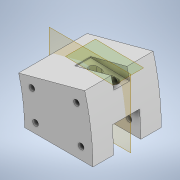
# Autodesk Inventor part: load_cell_mounting_block2
Saved by Autodesk Inventor 2022 (Build 260153000, 153)
## iProperties
Created: 2022-02-24
Part Number: load_cell_mounting_block2
Material: Generic
Document SubType Name: Modeling
Designer: Martijn
Density: 1 g/cm^3
Appearance: Default
Author: Martijn
Autodesk Inventor part; units mm, degrees
ref_plane "YZ Plane" through (0, 0, 0) normal (1, 0, 0) x (0, 1, 0)
ref_plane "XZ Plane" through (0, 0, 0) normal (0, 1, 0) x (-1, 0, 0)
ref_plane "XY Plane" through (0, 0, 0) normal (0, 0, 1) x (1, 0, 0)
sketch "Sketch1" plane through (0, 0, 0) normal (0, 0, 1) x (1, 0, 0)
  arc A0 (75, 0) -> (72.4444, 19.4114) centre (0, 0) ccw
  arc A1 (105, 0) -> (101.4222, 27.176) centre (0, 0) ccw
  line L0 (105, 0) -> (75, 0)
  line L1 (72.4444, 19.4114) -> (101.4222, 27.176)
  line L2 (75, 0) -> (0, 0)
  line L3 (0, 0) -> (72.4444, 19.4114)
  circle A2 centre (78.2518, 16.6329) radius 1.25
  circle A3 centre (79.8904, 4.1869) radius 1.25
  circle A4 centre (97.8148, 20.7912) radius 1.25
  circle A5 centre (99.863, 5.2336) radius 1.25
  line L4 (0, 0) -> (78.2518, 16.6329)
  line L5 (78.2518, 16.6329) -> (97.8148, 20.7912)
  line L6 (99.863, 5.2336) -> (79.8904, 4.1869)
  line L7 (79.8904, 4.1869) -> (0, 0)
  dimension "d0" = 20
  dimension "d1" = 15
  dimension "d2" = 3
  dimension "d3" = 3
  dimension "d4" = 2.5
  dimension "d5" = 80
  dimension "d6" = 75
  dimension "d7" = 105
  dimension "d8" = 80
  dimension "d9" = 20
  constraints: 16 end point, 6 centre point, 4 point on circle, 3 collinear, 3 equal radius, 2 coincident, 2 horizontal
  measures "d0" distance of L5.end L4.end
  measures "d1" angle of L0 L1
  measures "d2" angle of L1 L4
  measures "d3" angle of L0 L6
  measures "d4" diameter of A2
  measures "d5" distance of point (0, 0) L4.end
  measures "d6" radius of A0
  measures "d7" radius of A1
  measures "d8" distance of point (0, 0) L6.end
  measures "d9" distance of L6.end L6.start
extrude "Extrusion1" add sketch "Sketch1" along normal blind 30 contours A0 L1 A1 L0
ref_plane "Work Plane1" through (0, 0, 15) normal (0, 0, 1) x (1, 0, 0)
sketch "Sketch2" plane through (0, 0, 15) normal (0, 0, 1) x (1, 0, 0)
  line L0 (75, 0) -> (105, 0) projected
  line L1 (75, 0) -> (0, 0)
  line L2 (0, 0) -> (189.2794, -3.3039)
  line L3 (84.9871, -1.4835) -> (85.214, 11.5165)
  line L4 (85.214, 11.5165) -> (105.2109, 11.1675)
  line L5 (105.2109, 11.1675) -> (104.984, -1.8325)
  dimension "d12" = 13
  dimension "d13" = 1
  dimension "d14" = 85
  dimension "d15" = 105
  constraints: 10 end point, 2 parallel, 2 point on line, 1 horizontal, 1 perpendicular
  measures "d12" vertical distance of L3.start L3.end
  measures "d13" angle of L2 L0
  measures "d14" distance from line of L1.end L3
  measures "d15" distance from line of L5 L1.end
extrude "Extrusion2" cut sketch "Sketch2" along normal mid plane 12 contours L3 L4 L5 L2
sketch "Sketch3" plane through (104.4029, 11.1816, 9) normal (-0.0174524, -0.9998477, 0) x (0.9998477, -0.0174524, 0)
  arc A0 (-5, 4.3) -> (-5, 7.7) centre (-5, 6) ccw
  arc A1 (-7, 7.7) -> (-7, 4.3) centre (-7, 6) ccw
  line L0 (-7, 7.7) -> (-5, 7.7)
  line L1 (-5, 4.3) -> (-7, 4.3)
  line L2 (-19.1919, 12) -> (0.7921, 12) projected
  line L3 (0, 12) -> (0, 0) projected
  point P0 (-104.1919, -9)
  dimension "d19" = 3.4
  dimension "d20" = 6
  dimension "d21" = 5
  dimension "d22" = 2
  constraints: 4 end point, 4 point on circle, 4 tangent, 2 centre point, 2 horizontal
  measures "d19" distance between parallel lines of L1 L0
  measures "d20" distance from line of L2 A0.centre
  measures "d21" distance from line of L3 A0.centre
  measures "d22" distance of A0.centre A1.centre
extrude "Extrusion3" cut sketch "Sketch3" against normal blind 20
pattern_linear "Rectangular Pattern1" count 2 spacing 7.5 along (-0.9998477, 0.0174524, 0) of "Extrusion3"
ref_plane "Work Plane2" through (104.6822, 27.1792, 9) normal (-0.0174524, -0.9998477, 0) x (0.9998477, -0.0174524, 0)
sketch "Sketch5" plane through (104.6822, 27.1792, 9) normal (-0.0174524, -0.9998477, 0) x (0.9998477, -0.0174524, 0)
  line L0 (-19.0973, 2.5) -> (0.9027, 2.5)
  line L1 (0.9027, 2.5) -> (0.9027, 9.5)
  line L2 (0.9027, 9.5) -> (-19.0973, 9.5)
  line L3 (-19.0973, 9.5) -> (-19.0973, 2.5)
  line L4 (-3.2594, 21) -> (-32.0973, 21) projected
  line L5 (-32.0973, -9) -> (-32.0973, 21) projected
  point P0 (-104.1919, -9)
  point P1 (-19.0973, 6)
  dimension "d29" = 7
  dimension "d30" = 15
  dimension "d31" = 13
  dimension "d32" = 20
  constraints: 8 end point, 2 parallel, 1 horizontal, 1 midpoint, 1 perpendicular
  measures "d29" distance between parallel lines of L2 L0
  measures "d30" distance from line of L4 point (-19.097, 6)
  measures "d31" distance between parallel lines of L5 L3
  measures "d32" distance between parallel lines of L3 L1
extrude "Extrusion4" cut sketch "Sketch5" along normal blind 5
body "Solid1"
